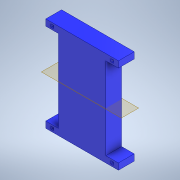
# Autodesk Inventor part: backplate
Saved by Autodesk Inventor 2020 (Build 240168000, 168)
## iProperties
Created: 2021-03-06
Part Number: backplate
Material: Generic
Document SubType Name: Modeling
Designer: Harry
Density: 1 g/cm^3
Appearance: Blue - Wall Paint - Glossy
Author: Harry
Autodesk Inventor part; units mm, degrees
ref_plane "YZ Plane" through (0, 0, 0) normal (1, 0, 0) x (0, 1, 0)
ref_plane "XZ Plane" through (0, 0, 0) normal (0, 1, 0) x (-1, 0, 0)
ref_plane "XY Plane" through (0, 0, 0) normal (0, 0, 1) x (1, 0, 0)
sketch "Sketch1" plane through (0, 0, 0) normal (0, 0, 1) x (1, 0, 0)
  line L0 (150, 300) -> (-150, 300)
  line L1 (-150, 300) -> (-150, -300)
  line L2 (-150, -300) -> (150, -300)
  line L3 (150, -300) -> (150, 300)
  line L4 (150, 300) -> (-150, -300) construction
  line L5 (-150, 300) -> (150, -300) construction
  point P0 (0, 0)
  dimension "d0" = 300
  dimension "d1" = 600
  constraints: 12 end point, 2 midpoint, 2 parallel, 1 horizontal, 1 perpendicular
  measures "d0" distance of L2.end L1.end
  measures "d1" distance of L1.end L0.end
extrude "Extrusion1" add sketch "Sketch1" along normal blind 100
sketch "Sketch2" plane through (0, 0, 100) normal (0, 0, 1) x (1, 0, 0)
  line L0 (-150, 300) -> (-150, -300) projected
  line L1 (-150, -300) -> (-230, -300)
  line L2 (-230, -300) -> (-230, -260)
  line L3 (-230, -260) -> (-150, -260)
  line L4 (-150, -260) -> (-150, -300)
  point P0 (0, 0)
  dimension "d4" = 80
  dimension "d5" = 40
  constraints: 8 end point, 2 parallel, 1 horizontal, 1 perpendicular
  measures "d4" distance of L2.end L3.end
  measures "d5" distance of L1.end L2.end
extrude "Extrusion2" add sketch "Sketch2" against normal up to surface (100 mm away)
sketch "Sketch3" plane through (0, 0, 100) normal (0, 0, 1) x (1, 0, 0)
  line L0 (-150, 300) -> (-150, -260) projected
  line L1 (-150, -260) -> (-150, -300) construction
  line L2 (150, -300) -> (-230, -300) projected
  line L3 (-150, -260) -> (-230, -260) projected
  line L4 (-230, -260) -> (-150, -300) construction
  line L5 (-150, -260) -> (-230, -300) construction
  line L6 (-182.2361, -289.15) -> (-197.7639, -289.15)
  line L7 (-197.7639, -289.15) -> (-197.7639, -270.85) construction
  line L8 (-197.7639, -270.85) -> (-182.2361, -270.85)
  line L9 (-182.2361, -289.15) -> (-197.7639, -270.85) construction
  line L10 (-197.7639, -289.15) -> (-182.2361, -270.85) construction
  arc A0 (-197.7639, -270.85) -> (-197.7639, -289.15) centre (-190, -280) ccw
  arc A1 (-182.2361, -289.15) -> (-182.2361, -270.85) centre (-190, -280) ccw
  point P0 (0, 0)
  dimension "d9" = 18.3
  constraints: 16 end point, 4 point on circle, 3 midpoint, 2 centre point, 1 horizontal, 1 parallel, 1 perpendicular, 1 point on line, 1 vertical
  measures "d9" distance of L6.end L7.end
extrude "Extrusion3" cut sketch "Sketch3" against normal up to surface (100 mm away)
ref_plane "Work Plane1" through (0, -300, 0) normal (1, 0, 0) x (0, 0, -1)
mirror "Mirror1" about plane through (0, -300, 0) normal (1, 0, 0) of "Extrusion2", "Extrusion3"
ref_plane "Work Plane2" through (-150, 0, 0) normal (0, 1, 0) x (1, 0, 0)
mirror "Mirror2" about plane through (-150, 0, 0) normal (0, 1, 0) of "Extrusion2", "Extrusion3", "Mirror1"
body "Solid1"
